Autodesk Fusion 360 part; units mm, degrees
(part 4 of 11)
  line L2513 (1.92, -15.2997) -> (1.92, -13.2625)
  arc A163 (1.92, -13.2625) -> (1.2372, -12.9797) centre (1.52, -13.2625) ccw
  line L2514 (1.2372, -12.9797) -> (-0.0459, -14.2627)
  line L2515 (-0.0459, -14.2627) -> (-0.0798, -14.2989)
  line L2516 (-0.0798, -14.2989) -> (-0.1133, -14.3397)
  line L2517 (-0.1133, -14.3397) -> (-0.1441, -14.3827)
  line L2518 (-0.1441, -14.3827) -> (-0.172, -14.4275)
  line L2519 (-0.172, -14.4275) -> (-0.1969, -14.4741)
  line L2520 (-0.1969, -14.4741) -> (-0.2187, -14.5222)
  line L2521 (-0.2187, -14.5222) -> (-0.2373, -14.5717)
  line L2522 (-0.2373, -14.5717) -> (-0.2526, -14.6222)
  line L2523 (-0.2526, -14.6222) -> (-0.2646, -14.6736)
  line L2524 (-0.2646, -14.6736) -> (-0.2732, -14.7258)
  line L2525 (-0.2732, -14.7258) -> (-0.2786, -14.7804)
  line L2526 (-0.2786, -14.7804) -> (-0.28, -14.8985)
  line L2527 (-0.28, -14.8985) -> (-0.28, -25.1009)
  line L2528 (-0.28, -25.1009) -> (-0.2786, -25.2189)
  line L2529 (-0.2786, -25.2189) -> (-0.2732, -25.2736)
  line L2530 (-0.2732, -25.2736) -> (-0.2646, -25.3257)
  line L2531 (-0.2646, -25.3257) -> (-0.2526, -25.3771)
  line L2532 (-0.2526, -25.3771) -> (-0.2373, -25.4277)
  line L2533 (-0.2373, -25.4277) -> (-0.2187, -25.4771)
  line L2534 (-0.2187, -25.4771) -> (-0.1969, -25.5252)
  line L2535 (-0.1969, -25.5252) -> (-0.172, -25.5718)
  line L2536 (-0.172, -25.5718) -> (-0.1441, -25.6166)
  line L2537 (-0.1441, -25.6166) -> (-0.1133, -25.6596)
  line L2538 (-0.1133, -25.6596) -> (-0.0798, -25.7004)
  line L2539 (-0.0798, -25.7004) -> (-0.0459, -25.7366)
  line L2540 (-0.0459, -25.7366) -> (1.2372, -27.0197)
  arc A164 (1.2372, -27.0197) -> (1.92, -26.7368) centre (1.52, -26.7368) ccw
  line L2541 (1.92, -26.7368) -> (1.92, -24.6997)
  line L2542 (1.92, -24.6997) -> (3.2765, -24.6997)
  line L2543 (3.2765, -24.6997) -> (5.82, -27.2432)
  line L2544 (5.82, -27.2432) -> (5.82, -29.8826)
  line L2545 (5.82, -29.8826) -> (5.937, -29.9997)
  line L2546 (5.937, -29.9997) -> (5.82, -30.1167)
  line L2547 (5.82, -30.1167) -> (5.82, -32.7562)
  line L2548 (5.82, -32.7562) -> (3.2765, -35.2997)
  line L2549 (3.2765, -35.2997) -> (1.92, -35.2997)
  line L2550 (1.92, -35.2997) -> (1.92, -33.2625)
  arc A165 (1.92, -33.2625) -> (1.2372, -32.9797) centre (1.52, -33.2625) ccw
  line L2551 (1.2372, -32.9797) -> (-0.0459, -34.2627)
  line L2552 (-0.0459, -34.2627) -> (-0.0798, -34.2989)
  line L2553 (-0.0798, -34.2989) -> (-0.1133, -34.3397)
  line L2554 (-0.1133, -34.3397) -> (-0.1441, -34.3827)
  line L2555 (-0.1441, -34.3827) -> (-0.172, -34.4275)
  line L2556 (-0.172, -34.4275) -> (-0.1969, -34.4741)
  line L2557 (-0.1969, -34.4741) -> (-0.2187, -34.5222)
  line L2558 (-0.2187, -34.5222) -> (-0.2373, -34.5717)
  line L2559 (-0.2373, -34.5717) -> (-0.2526, -34.6222)
  line L2560 (-0.2526, -34.6222) -> (-0.2646, -34.6736)
  line L2561 (-0.2646, -34.6736) -> (-0.2732, -34.7258)
  line L2562 (-0.2732, -34.7258) -> (-0.2786, -34.7804)
  line L2563 (-0.2786, -34.7804) -> (-0.28, -34.8985)
  line L2564 (-0.28, -34.8985) -> (-0.28, -45.1009)
  line L2565 (-0.28, -45.1009) -> (-0.2786, -45.2189)
  line L2566 (-0.2786, -45.2189) -> (-0.2732, -45.2736)
  line L2567 (-0.2732, -45.2736) -> (-0.2646, -45.3257)
  line L2568 (-0.2646, -45.3257) -> (-0.2526, -45.3771)
  line L2569 (-0.2526, -45.3771) -> (-0.2373, -45.4277)
  line L2570 (-0.2373, -45.4277) -> (-0.2187, -45.4771)
  line L2571 (-0.2187, -45.4771) -> (-0.1969, -45.5252)
  line L2572 (-0.1969, -45.5252) -> (-0.172, -45.5718)
  line L2573 (-0.172, -45.5718) -> (-0.1441, -45.6166)
  line L2574 (-0.1441, -45.6166) -> (-0.1133, -45.6596)
  line L2575 (-0.1133, -45.6596) -> (-0.0798, -45.7004)
  line L2576 (-0.0798, -45.7004) -> (-0.0459, -45.7366)
  line L2577 (-0.0459, -45.7366) -> (1.2372, -47.0197)
  arc A166 (1.2372, -47.0197) -> (1.92, -46.7368) centre (1.52, -46.7368) ccw
  line L2578 (1.92, -46.7368) -> (1.92, -44.6997)
  line L2579 (1.92, -44.6997) -> (3.2765, -44.6997)
  line L2580 (3.2765, -44.6997) -> (5.82, -47.2432)
  line L2581 (5.82, -47.2432) -> (5.82, -49.8826)
  line L2582 (5.82, -49.8826) -> (5.937, -49.9997)
  line L2583 (5.937, -49.9997) -> (5.82, -50.1167)
  line L2584 (5.82, -50.1167) -> (5.82, -52.7562)
  line L2585 (5.82, -52.7562) -> (3.2765, -55.2997)
  line L2586 (3.2765, -55.2997) -> (1.92, -55.2997)
  line L2587 (1.92, -55.2997) -> (1.92, -53.2625)
  arc A167 (1.92, -53.2625) -> (1.2372, -52.9797) centre (1.52, -53.2625) ccw
  line L2588 (1.2372, -52.9797) -> (-0.0459, -54.2627)
  line L2589 (-0.0459, -54.2627) -> (-0.0798, -54.2989)
  line L2590 (-0.0798, -54.2989) -> (-0.1133, -54.3397)
  line L2591 (-0.1133, -54.3397) -> (-0.1441, -54.3827)
  line L2592 (-0.1441, -54.3827) -> (-0.172, -54.4275)
  line L2593 (-0.172, -54.4275) -> (-0.1969, -54.4741)
  line L2594 (-0.1969, -54.4741) -> (-0.2187, -54.5222)
  line L2595 (-0.2187, -54.5222) -> (-0.2373, -54.5717)
  line L2596 (-0.2373, -54.5717) -> (-0.2526, -54.6222)
  line L2597 (-0.2526, -54.6222) -> (-0.2646, -54.6736)
  line L2598 (-0.2646, -54.6736) -> (-0.2732, -54.7258)
  line L2599 (-0.2732, -54.7258) -> (-0.2786, -54.7804)
  line L2600 (-0.2786, -54.7804) -> (-0.28, -54.8985)
  line L2601 (-0.28, -54.8985) -> (-0.28, -65.1009)
  line L2602 (-0.28, -65.1009) -> (-0.2786, -65.2189)
  line L2603 (-0.2786, -65.2189) -> (-0.2732, -65.2736)
  line L2604 (-0.2732, -65.2736) -> (-0.2646, -65.3257)
  line L2605 (-0.2646, -65.3257) -> (-0.2526, -65.3771)
  line L2606 (-0.2526, -65.3771) -> (-0.2373, -65.4277)
  line L2607 (-0.2373, -65.4277) -> (-0.2187, -65.4771)
  line L2608 (-0.2187, -65.4771) -> (-0.1969, -65.5252)
  line L2609 (-0.1969, -65.5252) -> (-0.172, -65.5718)
  line L2610 (-0.172, -65.5718) -> (-0.1441, -65.6166)
  line L2611 (-0.1441, -65.6166) -> (-0.1133, -65.6596)
  line L2612 (-0.1133, -65.6596) -> (-0.0798, -65.7004)
  line L2613 (-0.0798, -65.7004) -> (-0.0459, -65.7366)
  line L2614 (-0.0459, -65.7366) -> (1.2372, -67.0197)
  arc A168 (1.2372, -67.0197) -> (1.92, -66.7368) centre (1.52, -66.7368) ccw
  line L2615 (1.92, -66.7368) -> (1.92, -64.6997)
  line L2616 (1.92, -64.6997) -> (3.2765, -64.6997)
  line L2617 (3.2765, -64.6997) -> (5.82, -67.2432)
  line L2618 (5.82, -67.2432) -> (5.82, -69.8826)
  line L2619 (5.82, -69.8826) -> (5.937, -69.9997)
  line L2620 (5.937, -69.9997) -> (5.82, -70.1167)
  line L2621 (5.82, -70.1167) -> (5.82, -72.7562)
  line L2622 (5.82, -72.7562) -> (3.2765, -75.2997)
  line L2623 (3.2765, -75.2997) -> (1.92, -75.2997)
  line L2624 (1.92, -75.2997) -> (1.92, -73.2625)
  arc A169 (1.92, -73.2625) -> (1.2372, -72.9797) centre (1.52, -73.2625) ccw
  line L2625 (1.2372, -72.9797) -> (-0.0459, -74.2627)
  line L2626 (-0.0459, -74.2627) -> (-0.0798, -74.2989)
  line L2627 (-0.0798, -74.2989) -> (-0.1133, -74.3397)
  line L2628 (-0.1133, -74.3397) -> (-0.1441, -74.3827)
  line L2629 (-0.1441, -74.3827) -> (-0.172, -74.4275)
  line L2630 (-0.172, -74.4275) -> (-0.1969, -74.4741)
  line L2631 (-0.1969, -74.4741) -> (-0.2187, -74.5222)
  line L2632 (-0.2187, -74.5222) -> (-0.2373, -74.5717)
  line L2633 (-0.2373, -74.5717) -> (-0.2526, -74.6222)
  line L2634 (-0.2526, -74.6222) -> (-0.2646, -74.6736)
  line L2635 (-0.2646, -74.6736) -> (-0.2732, -74.7258)
  line L2636 (-0.2732, -74.7258) -> (-0.2786, -74.7804)
  line L2637 (-0.2786, -74.7804) -> (-0.28, -74.8985)
  line L2638 (-0.28, -74.8985) -> (-0.28, -78.4997)
  line L2639 (-0.28, -78.4997) -> (-0.28, -79.4997)
  arc A170 (-0.28, -79.4997) -> (0.42, -80.1997) centre (0.42, -79.4997) ccw
  line L2640 (0.42, -80.1997) -> (1.42, -80.1997)
  line L2641 (1.42, -80.1997) -> (5.0918, -80.1997)
  line L2642 (5.0918, -80.1997) -> (5.1413, -80.198)
  line L2643 (5.1413, -80.198) -> (5.1939, -80.1929)
  line L2644 (5.1939, -80.1929) -> (5.246, -80.1843)
  line L2645 (5.246, -80.1843) -> (5.2975, -80.1723)
  line L2646 (5.2975, -80.1723) -> (5.348, -80.1569)
  line L2647 (5.348, -80.1569) -> (5.3974, -80.1383)
  line L2648 (5.3974, -80.1383) -> (5.4455, -80.1165)
  line L2649 (5.4455, -80.1165) -> (5.4921, -80.0916)
  line L2650 (5.4921, -80.0916) -> (5.537, -80.0637)
  line L2651 (5.537, -80.0637) -> (5.5799, -80.033)
  line L2652 (5.5799, -80.033) -> (5.6207, -79.9995)
  line L2653 (5.6207, -79.9995) -> (5.6569, -79.9656)
  line L2654 (5.6569, -79.9656) -> (6.94, -78.6825)
  arc A171 (6.94, -78.6825) -> (6.6572, -77.9997) centre (6.6572, -78.3997) ccw
  line L2655 (6.6572, -77.9997) -> (4.62, -77.9997)
  line L2656 (4.62, -77.9997) -> (4.62, -76.6432)
  line L2657 (4.62, -76.6432) -> (7.1635, -74.0997)
  line L2658 (7.1635, -74.0997) -> (9.7981, -74.0997)
  line L2659 (9.7981, -74.0997) -> (9.9208, -73.977)
  line L2660 (9.9208, -73.977) -> (10.0448, -74.0997)
  line L2661 (10.0448, -74.0997) -> (12.6765, -74.0997)
  line L2662 (12.6765, -74.0997) -> (15.22, -76.6432)
  line L2663 (15.22, -76.6432) -> (15.22, -77.9997)
  line L2664 (15.22, -77.9997) -> (13.1828, -77.9997)
  arc A172 (13.1828, -77.9997) -> (12.9, -78.6825) centre (13.1828, -78.3997) ccw
  line L2665 (12.9, -78.6825) -> (14.1831, -79.9656)
  line L2666 (14.1831, -79.9656) -> (14.2193, -79.9995)
  line L2667 (14.2193, -79.9995) -> (14.2601, -80.033)
  line L2668 (14.2601, -80.033) -> (14.303, -80.0637)
  line L2669 (14.303, -80.0637) -> (14.3479, -80.0916)
  line L2670 (14.3479, -80.0916) -> (14.3945, -80.1165)
  line L2671 (14.3945, -80.1165) -> (14.4426, -80.1383)
  line L2672 (14.4426, -80.1383) -> (14.492, -80.1569)
  line L2673 (14.492, -80.1569) -> (14.5425, -80.1723)
  line L2674 (14.5425, -80.1723) -> (14.594, -80.1843)
  line L2675 (14.594, -80.1843) -> (14.6461, -80.1929)
  line L2676 (14.6461, -80.1929) -> (14.6987, -80.198)
  line L2677 (14.6987, -80.198) -> (14.7482, -80.1997)
  line L2678 (14.7482, -80.1997) -> (18.42, -80.1997)
  line L2679 (18.42, -80.1997) -> (19.42, -80.1997)
  arc A173 (19.42, -80.1997) -> (20.12, -79.4997) centre (19.42, -79.4997) ccw
  line L2680 (20.12, -79.4997) -> (20.12, -78.4997)
  line L2681 (20.12, -78.4997) -> (20.12, -74.8278)
  line L2682 (20.12, -74.8278) -> (20.1184, -74.7783)
  line L2683 (20.1184, -74.7783) -> (20.1132, -74.7258)
  line L2684 (20.1132, -74.7258) -> (20.1046, -74.6736)
  line L2685 (20.1046, -74.6736) -> (20.0926, -74.6222)
  line L2686 (20.0926, -74.6222) -> (20.0773, -74.5717)
  line L2687 (20.0773, -74.5717) -> (20.0587, -74.5222)
  line L2688 (20.0587, -74.5222) -> (20.0369, -74.4741)
  line L2689 (20.0369, -74.4741) -> (20.012, -74.4275)
  line L2690 (20.012, -74.4275) -> (19.9841, -74.3827)
  line L2691 (19.9841, -74.3827) -> (19.9533, -74.3397)
  line L2692 (19.9533, -74.3397) -> (19.9198, -74.2989)
  line L2693 (19.9198, -74.2989) -> (19.8859, -74.2627)
  line L2694 (19.8859, -74.2627) -> (18.6028, -72.9797)
  arc A174 (18.6028, -72.9797) -> (17.92, -73.2625) centre (18.32, -73.2625) ccw
  line L2695 (17.92, -73.2625) -> (17.92, -75.2997)
  line L2696 (17.92, -75.2997) -> (16.5635, -75.2997)
  line L2697 (16.5635, -75.2997) -> (14.02, -72.7562)
  line L2698 (14.02, -72.7562) -> (14.02, -70.1167)
  line L2699 (14.02, -70.1167) -> (13.903, -69.9997)
  line L2700 (13.903, -69.9997) -> (14.02, -69.8826)
  line L2701 (14.02, -69.8826) -> (14.02, -67.2432)
  line L2702 (14.02, -67.2432) -> (16.5635, -64.6997)
  line L2703 (16.5635, -64.6997) -> (17.92, -64.6997)
  line L2704 (17.92, -64.6997) -> (17.92, -66.7368)
  arc A175 (17.92, -66.7368) -> (18.6028, -67.0197) centre (18.32, -66.7368) ccw
  line L2705 (18.6028, -67.0197) -> (19.8859, -65.7366)
  line L2706 (19.8859, -65.7366) -> (19.9198, -65.7004)
  line L2707 (19.9198, -65.7004) -> (19.9533, -65.6596)
  line L2708 (19.9533, -65.6596) -> (19.9841, -65.6166)
  line L2709 (19.9841, -65.6166) -> (20.012, -65.5718)
  line L2710 (20.012, -65.5718) -> (20.0369, -65.5252)
  line L2711 (20.0369, -65.5252) -> (20.0587, -65.4771)
  line L2712 (20.0587, -65.4771) -> (20.0773, -65.4277)
  line L2713 (20.0773, -65.4277) -> (20.0926, -65.3771)
  line L2714 (20.0926, -65.3771) -> (20.1046, -65.3257)
  line L2715 (20.1046, -65.3257) -> (20.1132, -65.2736)
  line L2716 (20.1132, -65.2736) -> (20.1186, -65.2189)
  line L2717 (20.1186, -65.2189) -> (20.12, -65.1009)
  line L2718 (20.12, -65.1009) -> (20.12, -54.8985)
  line L2719 (20.12, -54.8985) -> (20.1186, -54.7804)
  line L2720 (20.1186, -54.7804) -> (20.1132, -54.7258)
  line L2721 (20.1132, -54.7258) -> (20.1046, -54.6736)
  line L2722 (20.1046, -54.6736) -> (20.0926, -54.6222)
  line L2723 (20.0926, -54.6222) -> (20.0773, -54.5717)
  line L2724 (20.0773, -54.5717) -> (20.0587, -54.5222)
  line L2725 (20.0587, -54.5222) -> (20.0369, -54.4741)
  line L2726 (20.0369, -54.4741) -> (20.012, -54.4275)
  line L2727 (20.012, -54.4275) -> (19.9841, -54.3827)
  line L2728 (19.9841, -54.3827) -> (19.9533, -54.3397)
  line L2729 (19.9533, -54.3397) -> (19.9198, -54.2989)
  line L2730 (19.9198, -54.2989) -> (19.8859, -54.2627)
  line L2731 (19.8859, -54.2627) -> (18.6028, -52.9797)
  arc A176 (18.6028, -52.9797) -> (17.92, -53.2625) centre (18.32, -53.2625) ccw
  line L2732 (17.92, -53.2625) -> (17.92, -55.2997)
  line L2733 (17.92, -55.2997) -> (16.5635, -55.2997)
  line L2734 (16.5635, -55.2997) -> (14.02, -52.7562)
  line L2735 (14.02, -52.7562) -> (14.02, -50.1167)
  line L2736 (14.02, -50.1167) -> (13.903, -49.9997)
  line L2737 (13.903, -49.9997) -> (14.02, -49.8826)
  line L2738 (14.02, -49.8826) -> (14.02, -47.2432)
  line L2739 (14.02, -47.2432) -> (16.5635, -44.6997)
  line L2740 (16.5635, -44.6997) -> (17.92, -44.6997)
  line L2741 (17.92, -44.6997) -> (17.92, -46.7368)
  arc A177 (17.92, -46.7368) -> (18.6028, -47.0197) centre (18.32, -46.7368) ccw
  line L2742 (18.6028, -47.0197) -> (19.8859, -45.7366)
  line L2743 (19.8859, -45.7366) -> (19.9198, -45.7004)
  line L2744 (19.9198, -45.7004) -> (19.9533, -45.6596)
  line L2745 (19.9533, -45.6596) -> (19.9841, -45.6166)
  line L2746 (19.9841, -45.6166) -> (20.012, -45.5718)
  line L2747 (20.012, -45.5718) -> (20.0369, -45.5252)
  line L2748 (20.0369, -45.5252) -> (20.0587, -45.4771)
  line L2749 (20.0587, -45.4771) -> (20.0773, -45.4277)
  line L2750 (20.0773, -45.4277) -> (20.0926, -45.3771)
  line L2751 (20.0926, -45.3771) -> (20.1046, -45.3257)
  line L2752 (20.1046, -45.3257) -> (20.1132, -45.2736)
  line L2753 (20.1132, -45.2736) -> (20.1186, -45.2189)
  line L2754 (20.1186, -45.2189) -> (20.12, -45.1009)
  line L2755 (20.12, -45.1009) -> (20.12, -34.8985)
  line L2756 (20.12, -34.8985) -> (20.1186, -34.7804)
  line L2757 (20.1186, -34.7804) -> (20.1132, -34.7258)
  line L2758 (20.1132, -34.7258) -> (20.1046, -34.6736)
  line L2759 (20.1046, -34.6736) -> (20.0926, -34.6222)
  line L2760 (20.0926, -34.6222) -> (20.0773, -34.5717)
  line L2761 (20.0773, -34.5717) -> (20.0587, -34.5222)
  line L2762 (20.0587, -34.5222) -> (20.0369, -34.4741)
  line L2763 (20.0369, -34.4741) -> (20.012, -34.4275)
  line L2764 (20.012, -34.4275) -> (19.9841, -34.3827)
  line L2765 (19.9841, -34.3827) -> (19.9533, -34.3397)
  line L2766 (19.9533, -34.3397) -> (19.9198, -34.2989)
  line L2767 (19.9198, -34.2989) -> (19.8859, -34.2627)
  line L2768 (19.8859, -34.2627) -> (18.6028, -32.9797)
  arc A178 (18.6028, -32.9797) -> (17.92, -33.2625) centre (18.32, -33.2625) ccw
  line L2769 (17.92, -33.2625) -> (17.92, -35.2997)
  line L2770 (17.92, -35.2997) -> (16.5635, -35.2997)
  line L2771 (16.5635, -35.2997) -> (14.02, -32.7562)
  line L2772 (14.02, -32.7562) -> (14.02, -30.1167)
  line L2773 (14.02, -30.1167) -> (13.903, -29.9997)
  line L2774 (13.903, -29.9997) -> (14.02, -29.8826)
  line L2775 (14.02, -29.8826) -> (14.02, -27.2432)
  line L2776 (14.02, -27.2432) -> (16.5635, -24.6997)
  line L2777 (16.5635, -24.6997) -> (17.92, -24.6997)
  line L2778 (17.92, -24.6997) -> (17.92, -26.7368)
  arc A179 (17.92, -26.7368) -> (18.6028, -27.0197) centre (18.32, -26.7368) ccw
  line L2779 (18.6028, -27.0197) -> (19.8859, -25.7366)
  line L2780 (19.8859, -25.7366) -> (19.9198, -25.7004)
  line L2781 (19.9198, -25.7004) -> (19.9533, -25.6596)
  line L2782 (19.9533, -25.6596) -> (19.9841, -25.6166)
  line L2783 (19.9841, -25.6166) -> (20.012, -25.5718)
  line L2784 (20.012, -25.5718) -> (20.0369, -25.5252)
  line L2785 (20.0369, -25.5252) -> (20.0587, -25.4771)
  line L2786 (20.0587, -25.4771) -> (20.0773, -25.4277)
  line L2787 (20.0773, -25.4277) -> (20.0926, -25.3771)
  line L2788 (20.0926, -25.3771) -> (20.1046, -25.3257)
  line L2789 (20.1046, -25.3257) -> (20.1132, -25.2736)
  line L2790 (20.1132, -25.2736) -> (20.1186, -25.2189)
  line L2791 (20.1186, -25.2189) -> (20.12, -25.1009)
  line L2792 (20.12, -25.1009) -> (20.12, -14.8985)
  line L2793 (20.12, -14.8985) -> (20.1186, -14.7804)
  line L2794 (20.1186, -14.7804) -> (20.1132, -14.7258)
  line L2795 (20.1132, -14.7258) -> (20.1046, -14.6736)
  line L2796 (20.1046, -14.6736) -> (20.0926, -14.6222)
  line L2797 (20.0926, -14.6222) -> (20.0773, -14.5717)
  line L2798 (20.0773, -14.5717) -> (20.0587, -14.5222)
  line L2799 (20.0587, -14.5222) -> (20.0369, -14.4741)
  line L2800 (20.0369, -14.4741) -> (20.012, -14.4275)
  line L2801 (20.012, -14.4275) -> (19.9841, -14.3827)
  line L2802 (19.9841, -14.3827) -> (19.9533, -14.3397)
  line L2803 (19.9533, -14.3397) -> (19.9198, -14.2989)
  line L2804 (19.9198, -14.2989) -> (19.8859, -14.2627)
  line L2805 (19.8859, -14.2627) -> (18.6028, -12.9797)
  arc A180 (18.6028, -12.9797) -> (17.92, -13.2625) centre (18.32, -13.2625) ccw
  line L2806 (17.92, -13.2625) -> (17.92, -15.2997)
  line L2807 (17.92, -15.2997) -> (16.5635, -15.2997)
  line L2808 (16.5635, -15.2997) -> (14.02, -12.7562)
  line L2809 (14.02, -12.7562) -> (14.02, -10.1167)
  line L2810 (14.02, -10.1167) -> (13.903, -9.9997)
  line L2811 (13.903, -9.9997) -> (14.02, -9.8826)
  line L2812 (14.02, -9.8826) -> (14.02, -7.2432)
  line L2813 (14.02, -7.2432) -> (16.5635, -4.6997)
  line L2814 (16.5635, -4.6997) -> (17.92, -4.6997)
  line L2815 (17.92, -4.6997) -> (17.92, -6.7368)
  arc A181 (17.92, -6.7368) -> (18.6028, -7.0197) centre (18.32, -6.7368) ccw
  line L2816 (18.6028, -7.0197) -> (19.8859, -5.7366)
  line L2817 (19.8859, -5.7366) -> (19.9198, -5.7004)
  line L2818 (9.92, -13.9755) -> (10.0441, -14.0997)
  line L2819 (10.0441, -14.0997) -> (12.6765, -14.0997)
  line L2820 (12.6765, -14.0997) -> (16.0765, -17.4997)
  line L2821 (16.0765, -17.4997) -> (17.92, -17.4997)
  line L2822 (17.92, -17.4997) -> (17.92, -22.4997)
  line L2823 (17.92, -22.4997) -> (16.0765, -22.4997)
  line L2824 (16.0765, -22.4997) -> (12.6765, -25.8997)
  line L2825 (12.6765, -25.8997) -> (10.0441, -25.8997)
  line L2826 (10.0441, -25.8997) -> (9.92, -26.0238)
  line L2827 (9.92, -26.0238) -> (9.7959, -25.8997)
  line L2828 (9.7959, -25.8997) -> (7.1635, -25.8997)
  line L2829 (7.1635, -25.8997) -> (3.7635, -22.4997)
  line L2830 (3.7635, -22.4997) -> (1.92, -22.4997)
  line L2831 (1.92, -22.4997) -> (1.92, -17.4997)
  line L2832 (1.92, -17.4997) -> (3.7635, -17.4997)
  line L2833 (3.7635, -17.4997) -> (7.1635, -14.0997)
  line L2834 (7.1635, -14.0997) -> (9.7959, -14.0997)
  line L2835 (9.7959, -14.0997) -> (9.92, -13.9755)
  line L2836 (9.92, -33.9755) -> (10.0441, -34.0997)
  line L2837 (10.0441, -34.0997) -> (12.6765, -34.0997)
  line L2838 (12.6765, -34.0997) -> (16.0765, -37.4997)
  line L2839 (16.0765, -37.4997) -> (17.92, -37.4997)
  line L2840 (17.92, -37.4997) -> (17.92, -42.4997)
  line L2841 (17.92, -42.4997) -> (16.0765, -42.4997)
  line L2842 (16.0765, -42.4997) -> (12.6765, -45.8997)
  line L2843 (12.6765, -45.8997) -> (10.0441, -45.8997)
  line L2844 (10.0441, -45.8997) -> (9.92, -46.0238)
  line L2845 (9.92, -46.0238) -> (9.7959, -45.8997)
  line L2846 (9.7959, -45.8997) -> (7.1635, -45.8997)
  line L2847 (7.1635, -45.8997) -> (3.7635, -42.4997)
  line L2848 (3.7635, -42.4997) -> (1.92, -42.4997)
  line L2849 (1.92, -42.4997) -> (1.92, -37.4997)
  line L2850 (1.92, -37.4997) -> (3.7635, -37.4997)
  line L2851 (3.7635, -37.4997) -> (7.1635, -34.0997)
  line L2852 (7.1635, -34.0997) -> (9.7959, -34.0997)
  line L2853 (9.7959, -34.0997) -> (9.92, -33.9755)
  line L2854 (16.0765, -57.4997) -> (17.92, -57.4997)
  line L2855 (17.92, -57.4997) -> (17.92, -62.4997)
  line L2856 (17.92, -62.4997) -> (16.0765, -62.4997)
  line L2857 (16.0765, -62.4997) -> (12.6765, -65.8997)
  line L2858 (12.6765, -65.8997) -> (10.0441, -65.8997)
  line L2859 (10.0441, -65.8997) -> (9.92, -66.0238)
  line L2860 (9.92, -66.0238) -> (9.7959, -65.8997)
  line L2861 (9.7959, -65.8997) -> (7.1635, -65.8997)
  line L2862 (7.1635, -65.8997) -> (3.7635, -62.4997)
  line L2863 (3.7635, -62.4997) -> (1.92, -62.4997)
  line L2864 (1.92, -62.4997) -> (1.92, -57.4997)
  line L2865 (1.92, -57.4997) -> (3.7635, -57.4997)
  line L2866 (3.7635, -57.4997) -> (7.1635, -54.0997)
  line L2867 (7.1635, -54.0997) -> (9.7959, -54.0997)
  line L2868 (9.7959, -54.0997) -> (9.92, -53.9755)
  line L2869 (9.92, -53.9755) -> (10.0441, -54.0997)
  line L2870 (10.0441, -54.0997) -> (12.6765, -54.0997)
  line L2871 (12.6765, -54.0997) -> (16.0765, -57.4997)
  line L2872 (9.92, -86.0238) -> (9.7959, -85.8997)
  line L2873 (9.7959, -85.8997) -> (7.1635, -85.8997)
  line L2874 (7.1635, -85.8997) -> (4.62, -83.3562)
  line L2875 (4.62, -83.3562) -> (4.62, -81.9997)
  line L2876 (4.62, -81.9997) -> (6.6572, -81.9997)
  arc A182 (6.6572, -81.9997) -> (6.94, -81.3168) centre (6.6572, -81.5997) ccw
  line L2877 (6.94, -81.3168) -> (5.6569, -80.0337)
  line L2878 (5.6569, -80.0337) -> (5.6207, -79.9999)
  line L2879 (5.6207, -79.9999) -> (5.5799, -79.9663)
  line L2880 (5.5799, -79.9663) -> (5.537, -79.9356)
  line L2881 (5.537, -79.9356) -> (5.4921, -79.9077)
  line L2882 (5.4921, -79.9077) -> (5.4455, -79.8828)
  line L2883 (5.4455, -79.8828) -> (5.3974, -79.861)
  line L2884 (5.3974, -79.861) -> (5.348, -79.8424)
  line L2885 (5.348, -79.8424) -> (5.2975, -79.8271)
  line L2886 (5.2975, -79.8271) -> (5.246, -79.8151)
  line L2887 (5.246, -79.8151) -> (5.1939, -79.8065)
  line L2888 (5.1939, -79.8065) -> (5.1413, -79.8013)
  line L2889 (5.1413, -79.8013) -> (5.0918, -79.7997)
  line L2890 (5.0918, -79.7997) -> (1.42, -79.7997)
  line L2891 (1.42, -79.7997) -> (0.42, -79.7997)
  arc A183 (0.42, -79.7997) -> (-0.28, -80.4997) centre (0.42, -80.4997) ccw
  line L2892 (-0.28, -80.4997) -> (-0.28, -81.4997)
  line L2893 (-0.28, -81.4997) -> (-0.28, -85.1009)
  line L2894 (-0.28, -85.1009) -> (-0.2786, -85.2189)
  line L2895 (-0.2786, -85.2189) -> (-0.2732, -85.2736)
  line L2896 (-0.2732, -85.2736) -> (-0.2646, -85.3257)
  line L2897 (-0.2646, -85.3257) -> (-0.2526, -85.3771)
  line L2898 (-0.2526, -85.3771) -> (-0.2373, -85.4277)
  line L2899 (-0.2373, -85.4277) -> (-0.2187, -85.4771)
  line L2900 (-0.2187, -85.4771) -> (-0.1969, -85.5252)
  line L2901 (-0.1969, -85.5252) -> (-0.172, -85.5718)
  line L2902 (-0.172, -85.5718) -> (-0.1441, -85.6166)
  line L2903 (-0.1441, -85.6166) -> (-0.1133, -85.6596)
  line L2904 (-0.1133, -85.6596) -> (-0.0798, -85.7004)
  line L2905 (-0.0798, -85.7004) -> (-0.0459, -85.7366)
  line L2906 (-0.0459, -85.7366) -> (1.2372, -87.0197)
  arc A184 (1.2372, -87.0197) -> (1.92, -86.7368) centre (1.52, -86.7368) ccw
  line L2907 (1.92, -86.7368) -> (1.92, -84.6997)
  line L2908 (1.92, -84.6997) -> (3.2765, -84.6997)
  line L2909 (3.2765, -84.6997) -> (5.82, -87.2432)
  line L2910 (5.82, -87.2432) -> (5.82, -89.8826)
  line L2911 (5.82, -89.8826) -> (5.937, -89.9997)
  line L2912 (5.937, -89.9997) -> (5.82, -90.1167)
  line L2913 (5.82, -90.1167) -> (5.82, -92.7562)
  line L2914 (5.82, -92.7562) -> (3.2765, -95.2997)
  line L2915 (3.2765, -95.2997) -> (1.92, -95.2997)
  line L2916 (1.92, -95.2997) -> (1.92, -93.2625)
  arc A185 (1.92, -93.2625) -> (1.2372, -92.9797) centre (1.52, -93.2625) ccw
  line L2917 (1.2372, -92.9797) -> (-0.0459, -94.2627)
  line L2918 (-0.0459, -94.2627) -> (-0.0798, -94.2989)
  line L2919 (-0.0798, -94.2989) -> (-0.1133, -94.3397)
  line L2920 (-0.1133, -94.3397) -> (-0.1441, -94.3827)
  line L2921 (-0.1441, -94.3827) -> (-0.172, -94.4275)
  line L2922 (-0.172, -94.4275) -> (-0.1969, -94.4741)
  line L2923 (-0.1969, -94.4741) -> (-0.2187, -94.5222)
  line L2924 (-0.2187, -94.5222) -> (-0.2373, -94.5717)
  line L2925 (-0.2373, -94.5717) -> (-0.2526, -94.6222)
  line L2926 (-0.2526, -94.6222) -> (-0.2646, -94.6736)
  line L2927 (-0.2646, -94.6736) -> (-0.2732, -94.7258)
  line L2928 (-0.2732, -94.7258) -> (-0.2786, -94.7804)
  line L2929 (-0.2786, -94.7804) -> (-0.28, -94.8985)
  line L2930 (-0.28, -94.8985) -> (-0.28, -105.1009)
  line L2931 (-0.28, -105.1009) -> (-0.2786, -105.2189)
  line L2932 (-0.2786, -105.2189) -> (-0.2732, -105.2736)
  line L2933 (-0.2732, -105.2736) -> (-0.2646, -105.3257)
  line L2934 (-0.2646, -105.3257) -> (-0.2526, -105.3771)
  line L2935 (-0.2526, -105.3771) -> (-0.2373, -105.4277)
  line L2936 (-0.2373, -105.4277) -> (-0.2187, -105.4771)
  line L2937 (-0.2187, -105.4771) -> (-0.1969, -105.5252)
  line L2938 (-0.1969, -105.5252) -> (-0.172, -105.5718)
  line L2939 (-0.172, -105.5718) -> (-0.1441, -105.6166)
  line L2940 (-0.1441, -105.6166) -> (-0.1133, -105.6596)
  line L2941 (-0.1133, -105.6596) -> (-0.0798, -105.7004)
  line L2942 (-0.0798, -105.7004) -> (-0.0459, -105.7366)
  line L2943 (-0.0459, -105.7366) -> (1.2372, -107.0197)
  arc A186 (1.2372, -107.0197) -> (1.92, -106.7368) centre (1.52, -106.7368) ccw
  line L2944 (1.92, -106.7368) -> (1.92, -104.6997)
  line L2945 (1.92, -104.6997) -> (3.2765, -104.6997)
  line L2946 (3.2765, -104.6997) -> (5.82, -107.2432)
  line L2947 (5.82, -107.2432) -> (5.82, -109.8826)
  line L2948 (5.82, -109.8826) -> (5.937, -109.9997)
  line L2949 (5.937, -109.9997) -> (5.82, -110.1167)
  line L2950 (5.82, -110.1167) -> (5.82, -112.7562)
  line L2951 (5.82, -112.7562) -> (3.2765, -115.2997)
  line L2952 (3.2765, -115.2997) -> (1.92, -115.2997)
  line L2953 (1.92, -115.2997) -> (1.92, -113.2625)
  arc A187 (1.92, -113.2625) -> (1.2372, -112.9797) centre (1.52, -113.2625) ccw
  line L2954 (1.2372, -112.9797) -> (-0.0459, -114.2627)
  line L2955 (-0.0459, -114.2627) -> (-0.0798, -114.2989)
  line L2956 (-0.0798, -114.2989) -> (-0.1133, -114.3397)
  line L2957 (-0.1133, -114.3397) -> (-0.1441, -114.3827)
  line L2958 (-0.1441, -114.3827) -> (-0.172, -114.4275)
  line L2959 (-0.172, -114.4275) -> (-0.1969, -114.4741)
  line L2960 (-0.1969, -114.4741) -> (-0.2187, -114.5222)
  line L2961 (-0.2187, -114.5222) -> (-0.2373, -114.5717)
  line L2962 (-0.2373, -114.5717) -> (-0.2526, -114.6222)
  line L2963 (-0.2526, -114.6222) -> (-0.2646, -114.6736)
  line L2964 (-0.2646, -114.6736) -> (-0.2732, -114.7258)
  line L2965 (-0.2732, -114.7258) -> (-0.2786, -114.7804)
  line L2966 (-0.2786, -114.7804) -> (-0.28, -114.8985)
  line L2967 (-0.28, -114.8985) -> (-0.28, -125.1009)
  line L2968 (-0.28, -125.1009) -> (-0.2786, -125.2189)
  line L2969 (-0.2786, -125.2189) -> (-0.2732, -125.2736)
  line L2970 (-0.2732, -125.2736) -> (-0.2646, -125.3257)
  line L2971 (-0.2646, -125.3257) -> (-0.2526, -125.3771)
  line L2972 (-0.2526, -125.3771) -> (-0.2373, -125.4277)
  line L2973 (-0.2373, -125.4277) -> (-0.2187, -125.4771)
  line L2974 (-0.2187, -125.4771) -> (-0.1969, -125.5252)
  line L2975 (-0.1969, -125.5252) -> (-0.172, -125.5718)
  line L2976 (-0.172, -125.5718) -> (-0.1441, -125.6166)
  line L2977 (-0.1441, -125.6166) -> (-0.1133, -125.6596)
  line L2978 (-0.1133, -125.6596) -> (-0.0798, -125.7004)
  line L2979 (-0.0798, -125.7004) -> (-0.0459, -125.7366)
  line L2980 (-0.0459, -125.7366) -> (1.2372, -127.0197)
  arc A188 (1.2372, -127.0197) -> (1.92, -126.7368) centre (1.52, -126.7368) ccw
  line L2981 (1.92, -126.7368) -> (1.92, -124.6997)
  line L2982 (1.92, -124.6997) -> (3.2765, -124.6997)
  line L2983 (3.2765, -124.6997) -> (5.82, -127.2432)
  line L2984 (5.82, -127.2432) -> (5.82, -129.8826)
  line L2985 (5.82, -129.8826) -> (5.937, -129.9997)
  line L2986 (5.937, -129.9997) -> (5.82, -130.1167)
  line L2987 (5.82, -130.1167) -> (5.82, -132.7562)
  line L2988 (5.82, -132.7562) -> (3.2765, -135.2997)
  line L2989 (3.2765, -135.2997) -> (1.92, -135.2997)
  line L2990 (1.92, -135.2997) -> (1.92, -133.2625)
  arc A189 (1.92, -133.2625) -> (1.2372, -132.9797) centre (1.52, -133.2625) ccw
  line L2991 (1.2372, -132.9797) -> (-0.0459, -134.2627)
  line L2992 (-0.0459, -134.2627) -> (-0.0798, -134.2989)
  line L2993 (-0.0798, -134.2989) -> (-0.1133, -134.3397)
  line L2994 (-0.1133, -134.3397) -> (-0.1441, -134.3827)
  line L2995 (-0.1441, -134.3827) -> (-0.172, -134.4275)
  line L2996 (-0.172, -134.4275) -> (-0.1969, -134.4741)
  line L2997 (-0.1969, -134.4741) -> (-0.2187, -134.5222)
  line L2998 (-0.2187, -134.5222) -> (-0.2373, -134.5717)
  line L2999 (-0.2373, -134.5717) -> (-0.2526, -134.6222)
  line L3000 (-0.2526, -134.6222) -> (-0.2646, -134.6736)
  line L3001 (-0.2646, -134.6736) -> (-0.2732, -134.7258)
  line L3002 (-0.2732, -134.7258) -> (-0.2786, -134.7804)
  line L3003 (-0.2786, -134.7804) -> (-0.28, -134.8985)
  line L3004 (-0.28, -134.8985) -> (-0.28, -138.4997)
  line L3005 (-0.28, -138.4997) -> (-0.28, -139.4997)
  arc A190 (-0.28, -139.4997) -> (0.42, -140.1997) centre (0.42, -139.4997) ccw
  line L3006 (0.42, -140.1997) -> (1.42, -140.1997)
  line L3007 (1.42, -140.1997) -> (5.0918, -140.1997)
  line L3008 (5.0918, -140.1997) -> (5.1413, -140.198)
  line L3009 (5.1413, -140.198) -> (5.1939, -140.1929)
  line L3010 (5.1939, -140.1929) -> (5.246, -140.1843)
  line L3011 (5.246, -140.1843) -> (5.2975, -140.1723)
  line L3012 (5.2975, -140.1723) -> (5.348, -140.1569)
  line L3013 (5.348, -140.1569) -> (5.3974, -140.1383)
  line L3014 (5.3974, -140.1383) -> (5.4455, -140.1165)
  line L3015 (5.4455, -140.1165) -> (5.4921, -140.0916)
  line L3016 (5.4921, -140.0916) -> (5.537, -140.0637)
  line L3017 (5.537, -140.0637) -> (5.5799, -140.033)
  line L3018 (5.5799, -140.033) -> (5.6207, -139.9995)
  line L3019 (5.6207, -139.9995) -> (5.6569, -139.9656)
  line L3020 (5.6569, -139.9656) -> (6.94, -138.6825)
  arc A191 (6.94, -138.6825) -> (6.6572, -137.9997) centre (6.6572, -138.3997) ccw
  line L3021 (6.6572, -137.9997) -> (4.62, -137.9997)
  line L3022 (4.62, -137.9997) -> (4.62, -136.6432)
  line L3023 (4.62, -136.6432) -> (7.1635, -134.0997)
  line L3024 (7.1635, -134.0997) -> (9.7981, -134.0997)
  line L3025 (9.7981, -134.0997) -> (9.9208, -133.977)
  line L3026 (9.9208, -133.977) -> (10.0448, -134.0997)
  line L3027 (10.0448, -134.0997) -> (12.6765, -134.0997)
  line L3028 (12.6765, -134.0997) -> (15.22, -136.6432)
  line L3029 (15.22, -136.6432) -> (15.22, -137.9997)
  line L3030 (15.22, -137.9997) -> (13.1828, -137.9997)
  arc A192 (13.1828, -137.9997) -> (12.9, -138.6825) centre (13.1828, -138.3997) ccw
  line L3031 (12.9, -138.6825) -> (14.1831, -139.9656)
  line L3032 (14.1831, -139.9656) -> (14.2193, -139.9995)
  line L3033 (14.2193, -139.9995) -> (14.2601, -140.033)
  line L3034 (14.2601, -140.033) -> (14.303, -140.0637)
  line L3035 (14.303, -140.0637) -> (14.3479, -140.0916)
  line L3036 (14.3479, -140.0916) -> (14.3945, -140.1165)
  line L3037 (14.3945, -140.1165) -> (14.4426, -140.1383)
  line L3038 (14.4426, -140.1383) -> (14.492, -140.1569)
  line L3039 (14.492, -140.1569) -> (14.5425, -140.1723)
  line L3040 (14.5425, -140.1723) -> (14.594, -140.1843)
  line L3041 (14.594, -140.1843) -> (14.6461, -140.1929)
  line L3042 (14.6461, -140.1929) -> (14.6987, -140.198)
  line L3043 (14.6987, -140.198) -> (14.7482, -140.1997)
  line L3044 (14.7482, -140.1997) -> (18.42, -140.1997)
  line L3045 (18.42, -140.1997) -> (19.42, -140.1997)
  arc A193 (19.42, -140.1997) -> (20.12, -139.4997) centre (19.42, -139.4997) ccw
  line L3046 (20.12, -139.4997) -> (20.12, -138.4997)
  line L3047 (20.12, -138.4997) -> (20.12, -134.8278)
  line L3048 (20.12, -134.8278) -> (20.1184, -134.7783)
  line L3049 (20.1184, -134.7783) -> (20.1132, -134.7258)
  line L3050 (20.1132, -134.7258) -> (20.1046, -134.6736)
  line L3051 (20.1046, -134.6736) -> (20.0926, -134.6222)
  line L3052 (20.0926, -134.6222) -> (20.0773, -134.5717)
  line L3053 (20.0773, -134.5717) -> (20.0587, -134.5222)
  line L3054 (20.0587, -134.5222) -> (20.0369, -134.4741)
  line L3055 (20.0369, -134.4741) -> (20.012, -134.4275)
  line L3056 (20.012, -134.4275) -> (19.9841, -134.3827)
  line L3057 (19.9841, -134.3827) -> (19.9533, -134.3397)
  line L3058 (19.9533, -134.3397) -> (19.9198, -134.2989)
  line L3059 (19.9198, -134.2989) -> (19.8859, -134.2627)
  line L3060 (19.8859, -134.2627) -> (18.6028, -132.9797)
  arc A194 (18.6028, -132.9797) -> (17.92, -133.2625) centre (18.32, -133.2625) ccw
  line L3061 (17.92, -133.2625) -> (17.92, -135.2997)
  line L3062 (17.92, -135.2997) -> (16.5635, -135.2997)
  line L3063 (16.5635, -135.2997) -> (14.02, -132.7562)
  line L3064 (14.02, -132.7562) -> (14.02, -130.1167)
  line L3065 (14.02, -130.1167) -> (13.903, -129.9997)
  line L3066 (13.903, -129.9997) -> (14.02, -129.8826)
  line L3067 (14.02, -129.8826) -> (14.02, -127.2432)
  line L3068 (14.02, -127.2432) -> (16.5635, -124.6997)
  line L3069 (16.5635, -124.6997) -> (17.92, -124.6997)
  line L3070 (17.92, -124.6997) -> (17.92, -126.7368)
  arc A195 (17.92, -126.7368) -> (18.6028, -127.0197) centre (18.32, -126.7368) ccw
  line L3071 (18.6028, -127.0197) -> (19.8859, -125.7366)
  line L3072 (19.8859, -125.7366) -> (19.9198, -125.7004)
  line L3073 (19.9198, -125.7004) -> (19.9533, -125.6596)
  line L3074 (19.9533, -125.6596) -> (19.9841, -125.6166)
  line L3075 (19.9841, -125.6166) -> (20.012, -125.5718)
  line L3076 (20.012, -125.5718) -> (20.0369, -125.5252)
  line L3077 (20.0369, -125.5252) -> (20.0587, -125.4771)
  line L3078 (20.0587, -125.4771) -> (20.0773, -125.4277)
  line L3079 (20.0773, -125.4277) -> (20.0926, -125.3771)
  line L3080 (20.0926, -125.3771) -> (20.1046, -125.3257)
  line L3081 (20.1046, -125.3257) -> (20.1132, -125.2736)
  line L3082 (20.1132, -125.2736) -> (20.1186, -125.2189)
  line L3083 (20.1186, -125.2189) -> (20.12, -125.1009)
  line L3084 (20.12, -125.1009) -> (20.12, -114.8985)
  line L3085 (20.12, -114.8985) -> (20.1186, -114.7804)
  line L3086 (20.1186, -114.7804) -> (20.1132, -114.7258)
  line L3087 (20.1132, -114.7258) -> (20.1046, -114.6736)
  line L3088 (20.1046, -114.6736) -> (20.0926, -114.6222)
  line L3089 (20.0926, -114.6222) -> (20.0773, -114.5717)
  line L3090 (20.0773, -114.5717) -> (20.0587, -114.5222)
  line L3091 (20.0587, -114.5222) -> (20.0369, -114.4741)
  line L3092 (20.0369, -114.4741) -> (20.012, -114.4275)
  line L3093 (20.012, -114.4275) -> (19.9841, -114.3827)
  line L3094 (19.9841, -114.3827) -> (19.9533, -114.3397)
  line L3095 (19.9533, -114.3397) -> (19.9198, -114.2989)
  line L3096 (19.9198, -114.2989) -> (19.8859, -114.2627)
  line L3097 (19.8859, -114.2627) -> (18.6028, -112.9797)
  arc A196 (18.6028, -112.9797) -> (17.92, -113.2625) centre (18.32, -113.2625) ccw
  line L3098 (17.92, -113.2625) -> (17.92, -115.2997)
  line L3099 (17.92, -115.2997) -> (16.5635, -115.2997)
  line L3100 (16.5635, -115.2997) -> (14.02, -112.7562)
  line L3101 (14.02, -112.7562) -> (14.02, -110.1167)
  line L3102 (14.02, -110.1167) -> (13.903, -109.9997)
  line L3103 (13.903, -109.9997) -> (14.02, -109.8826)
  line L3104 (14.02, -109.8826) -> (14.02, -107.2432)
  line L3105 (14.02, -107.2432) -> (16.5635, -104.6997)
  line L3106 (16.5635, -104.6997) -> (17.92, -104.6997)
  line L3107 (17.92, -104.6997) -> (17.92, -106.7368)
  arc A197 (17.92, -106.7368) -> (18.6028, -107.0197) centre (18.32, -106.7368) ccw
  line L3108 (18.6028, -107.0197) -> (19.8859, -105.7366)
  line L3109 (19.8859, -105.7366) -> (19.9198, -105.7004)
  line L3110 (19.9198, -105.7004) -> (19.9533, -105.6596)
  line L3111 (19.9533, -105.6596) -> (19.9841, -105.6166)
  line L3112 (19.9841, -105.6166) -> (20.012, -105.5718)
  line L3113 (20.012, -105.5718) -> (20.0369, -105.5252)
  line L3114 (20.0369, -105.5252) -> (20.0587, -105.4771)
  line L3115 (20.0587, -105.4771) -> (20.0773, -105.4277)
  line L3116 (20.0773, -105.4277) -> (20.0926, -105.3771)
  line L3117 (20.0926, -105.3771) -> (20.1046, -105.3257)
  line L3118 (20.1046, -105.3257) -> (20.1132, -105.2736)
  line L3119 (20.1132, -105.2736) -> (20.1186, -105.2189)
  line L3120 (20.1186, -105.2189) -> (20.12, -105.1009)
  line L3121 (20.12, -105.1009) -> (20.12, -94.8985)
  line L3122 (20.12, -94.8985) -> (20.1186, -94.7804)
  line L3123 (20.1186, -94.7804) -> (20.1132, -94.7258)
  line L3124 (20.1132, -94.7258) -> (20.1046, -94.6736)
  line L3125 (20.1046, -94.6736) -> (20.0926, -94.6222)
  line L3126 (20.0926, -94.6222) -> (20.0773, -94.5717)
  line L3127 (20.0773, -94.5717) -> (20.0587, -94.5222)
  line L3128 (20.0587, -94.5222) -> (20.0369, -94.4741)
  line L3129 (20.0369, -94.4741) -> (20.012, -94.4275)
  line L3130 (20.012, -94.4275) -> (19.9841, -94.3827)
  line L3131 (19.9841, -94.3827) -> (19.9533, -94.3397)
  line L3132 (19.9533, -94.3397) -> (19.9198, -94.2989)
  line L3133 (19.9198, -94.2989) -> (19.8859, -94.2627)
  line L3134 (19.8859, -94.2627) -> (18.6028, -92.9797)
  arc A198 (18.6028, -92.9797) -> (17.92, -93.2625) centre (18.32, -93.2625) ccw
  line L3135 (17.92, -93.2625) -> (17.92, -95.2997)
  line L3136 (17.92, -95.2997) -> (16.5635, -95.2997)
  line L3137 (16.5635, -95.2997) -> (14.02, -92.7562)
  line L3138 (14.02, -92.7562) -> (14.02, -90.1167)
  line L3139 (14.02, -90.1167) -> (13.903, -89.9997)
  line L3140 (13.903, -89.9997) -> (14.02, -89.8826)
  line L3141 (14.02, -89.8826) -> (14.02, -87.2432)
  line L3142 (14.02, -87.2432) -> (16.5635, -84.6997)
  line L3143 (16.5635, -84.6997) -> (17.92, -84.6997)
  line L3144 (17.92, -84.6997) -> (17.92, -86.7368)
  arc A199 (17.92, -86.7368) -> (18.6028, -87.0197) centre (18.32, -86.7368) ccw
  line L3145 (18.6028, -87.0197) -> (19.8859, -85.7366)
  line L3146 (19.8859, -85.7366) -> (19.9198, -85.7004)
  line L3147 (19.9198, -85.7004) -> (19.9533, -85.6596)
  line L3148 (19.9533, -85.6596) -> (19.9841, -85.6166)
  line L3149 (19.9841, -85.6166) -> (20.012, -85.5718)
  line L3150 (20.012, -85.5718) -> (20.0369, -85.5252)
  line L3151 (20.0369, -85.5252) -> (20.0587, -85.4771)
  line L3152 (20.0587, -85.4771) -> (20.0773, -85.4277)
  line L3153 (20.0773, -85.4277) -> (20.0926, -85.3771)
  line L3154 (20.0926, -85.3771) -> (20.1046, -85.3257)
  line L3155 (20.1046, -85.3257) -> (20.1132, -85.2736)
  line L3156 (20.1132, -85.2736) -> (20.1184, -85.221)
  line L3157 (20.1184, -85.221) -> (20.12, -85.1715)
  line L3158 (20.12, -85.1715) -> (20.12, -81.4997)
  line L3159 (20.12, -81.4997) -> (20.12, -80.4997)
  arc A200 (20.12, -80.4997) -> (19.42, -79.7997) centre (19.42, -80.4997) ccw
  line L3160 (19.42, -79.7997) -> (18.42, -79.7997)
  line L3161 (18.42, -79.7997) -> (14.7482, -79.7997)
  line L3162 (14.7482, -79.7997) -> (14.6987, -79.8013)
  line L3163 (14.6987, -79.8013) -> (14.6461, -79.8065)
  line L3164 (14.6461, -79.8065) -> (14.594, -79.8151)
  line L3165 (14.594, -79.8151) -> (14.5425, -79.8271)
  line L3166 (14.5425, -79.8271) -> (14.492, -79.8424)
  line L3167 (14.492, -79.8424) -> (14.4426, -79.861)
  line L3168 (14.4426, -79.861) -> (14.3945, -79.8828)
  line L3169 (14.3945, -79.8828) -> (14.3479, -79.9077)
  line L3170 (14.3479, -79.9077) -> (14.303, -79.9356)
  line L3171 (14.303, -79.9356) -> (14.2601, -79.9663)
  line L3172 (14.2601, -79.9663) -> (14.2193, -79.9999)
  line L3173 (14.2193, -79.9999) -> (14.1831, -80.0337)
  line L3174 (14.1831, -80.0337) -> (12.9, -81.3168)
  arc A201 (12.9, -81.3168) -> (13.1828, -81.9997) centre (13.1828, -81.5997) ccw
  line L3175 (13.1828, -81.9997) -> (15.22, -81.9997)
  line L3176 (15.22, -81.9997) -> (15.22, -83.3562)
  line L3177 (15.22, -83.3562) -> (12.6765, -85.8997)
  line L3178 (12.6765, -85.8997) -> (10.0441, -85.8997)
  line L3179 (10.0441, -85.8997) -> (9.92, -86.0238)
  line L3180 (16.0765, -97.4997) -> (17.92, -97.4997)
  line L3181 (17.92, -97.4997) -> (17.92, -102.4997)
  line L3182 (17.92, -102.4997) -> (16.0765, -102.4997)
  line L3183 (16.0765, -102.4997) -> (12.6765, -105.8997)
  line L3184 (12.6765, -105.8997) -> (10.0441, -105.8997)
  line L3185 (10.0441, -105.8997) -> (9.92, -106.0238)
  line L3186 (9.92, -106.0238) -> (9.7959, -105.8997)
  line L3187 (9.7959, -105.8997) -> (7.1635, -105.8997)
  line L3188 (7.1635, -105.8997) -> (3.7635, -102.4997)
  line L3189 (3.7635, -102.4997) -> (1.92, -102.4997)
  line L3190 (1.92, -102.4997) -> (1.92, -97.4997)
  line L3191 (1.92, -97.4997) -> (3.7635, -97.4997)
  line L3192 (3.7635, -97.4997) -> (7.1635, -94.0997)
  line L3193 (7.1635, -94.0997) -> (9.7959, -94.0997)
  line L3194 (9.7959, -94.0997) -> (9.92, -93.9755)
  line L3195 (9.92, -93.9755) -> (10.0441, -94.0997)
  line L3196 (10.0441, -94.0997) -> (12.6765, -94.0997)
  line L3197 (12.6765, -94.0997) -> (16.0765, -97.4997)
  line L3198 (9.92, -113.9755) -> (10.0441, -114.0997)
  line L3199 (10.0441, -114.0997) -> (12.6765, -114.0997)
  line L3200 (12.6765, -114.0997) -> (16.0765, -117.4997)
  line L3201 (16.0765, -117.4997) -> (17.92, -117.4997)
  line L3202 (17.92, -117.4997) -> (17.92, -122.4997)
  line L3203 (17.92, -122.4997) -> (16.0765, -122.4997)
  line L3204 (16.0765, -122.4997) -> (12.6765, -125.8997)
  line L3205 (12.6765, -125.8997) -> (10.0441, -125.8997)
  line L3206 (10.0441, -125.8997) -> (9.92, -126.0238)
  line L3207 (9.92, -126.0238) -> (9.7959, -125.8997)
  line L3208 (9.7959, -125.8997) -> (7.1635, -125.8997)
  line L3209 (7.1635, -125.8997) -> (3.7635, -122.4997)
  line L3210 (3.7635, -122.4997) -> (1.92, -122.4997)
  line L3211 (1.92, -122.4997) -> (1.92, -117.4997)
  line L3212 (1.92, -117.4997) -> (3.7635, -117.4997)
  line L3213 (3.7635, -117.4997) -> (7.1635, -114.0997)
  line L3214 (7.1635, -114.0997) -> (9.7959, -114.0997)
  line L3215 (9.7959, -114.0997) -> (9.92, -113.9755)
  line L3216 (-0.2786, -145.2189) -> (-0.2732, -145.2736)
  line L3217 (-0.2732, -145.2736) -> (-0.2646, -145.3257)
  line L3218 (-0.2646, -145.3257) -> (-0.2526, -145.3771)
  line L3219 (-0.2526, -145.3771) -> (-0.2373, -145.4277)
  line L3220 (-0.2373, -145.4277) -> (-0.2187, -145.4771)
  line L3221 (-0.2187, -145.4771) -> (-0.1969, -145.5252)
  line L3222 (-0.1969, -145.5252) -> (-0.172, -145.5718)
  line L3223 (-0.172, -145.5718) -> (-0.1441, -145.6166)
  line L3224 (-0.1441, -145.6166) -> (-0.1133, -145.6596)
  line L3225 (-0.1133, -145.6596) -> (-0.0798, -145.7004)
  line L3226 (-0.0798, -145.7004) -> (-0.0459, -145.7366)
  line L3227 (-0.0459, -145.7366) -> (1.2372, -147.0197)
  arc A202 (1.2372, -147.0197) -> (1.92, -146.7368) centre (1.52, -146.7368) ccw
  line L3228 (1.92, -146.7368) -> (1.92, -144.6997)
  line L3229 (1.92, -144.6997) -> (3.2765, -144.6997)
  line L3230 (3.2765, -144.6997) -> (5.82, -147.2432)
  line L3231 (5.82, -147.2432) -> (5.82, -149.8826)
  line L3232 (5.82, -149.8826) -> (5.937, -149.9997)
  line L3233 (5.937, -149.9997) -> (5.82, -150.1167)
  line L3234 (5.82, -150.1167) -> (5.82, -152.7562)
  line L3235 (5.82, -152.7562) -> (3.2765, -155.2997)
  line L3236 (3.2765, -155.2997) -> (1.92, -155.2997)
  line L3237 (1.92, -155.2997) -> (1.92, -153.2625)
  arc A203 (1.92, -153.2625) -> (1.2372, -152.9797) centre (1.52, -153.2625) ccw
  line L3238 (1.2372, -152.9797) -> (-0.0459, -154.2627)
  line L3239 (-0.0459, -154.2627) -> (-0.0798, -154.2989)
  line L3240 (-0.0798, -154.2989) -> (-0.1133, -154.3397)
  line L3241 (-0.1133, -154.3397) -> (-0.1441, -154.3827)
  line L3242 (-0.1441, -154.3827) -> (-0.172, -154.4275)
  line L3243 (-0.172, -154.4275) -> (-0.1969, -154.4741)
  line L3244 (-0.1969, -154.4741) -> (-0.2187, -154.5222)
  line L3245 (-0.2187, -154.5222) -> (-0.2373, -154.5717)
  line L3246 (-0.2373, -154.5717) -> (-0.2526, -154.6222)
  line L3247 (-0.2526, -154.6222) -> (-0.2646, -154.6736)
  line L3248 (-0.2646, -154.6736) -> (-0.2732, -154.7258)
  line L3249 (-0.2732, -154.7258) -> (-0.2786, -154.7804)
  line L3250 (-0.2786, -154.7804) -> (-0.28, -154.8985)
  line L3251 (-0.28, -154.8985) -> (-0.28, -165.1009)
  line L3252 (-0.28, -165.1009) -> (-0.2786, -165.2189)
  line L3253 (-0.2786, -165.2189) -> (-0.2732, -165.2736)
  line L3254 (-0.2732, -165.2736) -> (-0.2646, -165.3257)
  line L3255 (-0.2646, -165.3257) -> (-0.2526, -165.3771)
  line L3256 (-0.2526, -165.3771) -> (-0.2373, -165.4277)
  line L3257 (-0.2373, -165.4277) -> (-0.2187, -165.4771)
  line L3258 (-0.2187, -165.4771) -> (-0.1969, -165.5252)
  line L3259 (-0.1969, -165.5252) -> (-0.172, -165.5718)
  line L3260 (-0.172, -165.5718) -> (-0.1441, -165.6166)
  line L3261 (-0.1441, -165.6166) -> (-0.1133, -165.6596)
  line L3262 (-0.1133, -165.6596) -> (-0.0798, -165.7004)
  line L3263 (-0.0798, -165.7004) -> (-0.0459, -165.7366)
  line L3264 (-0.0459, -165.7366) -> (1.2372, -167.0197)
  arc A204 (1.2372, -167.0197) -> (1.92, -166.7368) centre (1.52, -166.7368) ccw
  line L3265 (1.92, -166.7368) -> (1.92, -164.6997)
  line L3266 (1.92, -164.6997) -> (3.2765, -164.6997)
  line L3267 (3.2765, -164.6997) -> (5.82, -167.2432)
  line L3268 (5.82, -167.2432) -> (5.82, -169.8826)
  line L3269 (5.82, -169.8826) -> (5.937, -169.9997)
  line L3270 (5.937, -169.9997) -> (5.82, -170.1167)
  line L3271 (5.82, -170.1167) -> (5.82, -172.7562)
  line L3272 (5.82, -172.7562) -> (3.2765, -175.2997)
  line L3273 (3.2765, -175.2997) -> (1.92, -175.2997)
  line L3274 (1.92, -175.2997) -> (1.92, -173.2625)
  arc A205 (1.92, -173.2625) -> (1.2372, -172.9797) centre (1.52, -173.2625) ccw
  line L3275 (1.2372, -172.9797) -> (-0.0459, -174.2627)
  line L3276 (-0.0459, -174.2627) -> (-0.0798, -174.2989)
  line L3277 (-0.0798, -174.2989) -> (-0.1133, -174.3397)
  line L3278 (-0.1133, -174.3397) -> (-0.1441, -174.3827)
  line L3279 (-0.1441, -174.3827) -> (-0.172, -174.4275)
  line L3280 (-0.172, -174.4275) -> (-0.1969, -174.4741)
  line L3281 (-0.1969, -174.4741) -> (-0.2187, -174.5222)
  line L3282 (-0.2187, -174.5222) -> (-0.2373, -174.5717)
  line L3283 (-0.2373, -174.5717) -> (-0.2526, -174.6222)
  line L3284 (-0.2526, -174.6222) -> (-0.2646, -174.6736)
  line L3285 (-0.2646, -174.6736) -> (-0.2732, -174.7258)
  line L3286 (-0.2732, -174.7258) -> (-0.2786, -174.7804)
  line L3287 (-0.2786, -174.7804) -> (-0.28, -174.8985)
  line L3288 (-0.28, -174.8985) -> (-0.28, -185.1009)
  line L3289 (-0.28, -185.1009) -> (-0.2786, -185.2189)
  line L3290 (-0.2786, -185.2189) -> (-0.2732, -185.2736)
  line L3291 (-0.2732, -185.2736) -> (-0.2646, -185.3257)
  line L3292 (-0.2646, -185.3257) -> (-0.2526, -185.3771)
  line L3293 (-0.2526, -185.3771) -> (-0.2373, -185.4277)
  line L3294 (-0.2373, -185.4277) -> (-0.2187, -185.4771)
  line L3295 (-0.2187, -185.4771) -> (-0.1969, -185.5252)
  line L3296 (-0.1969, -185.5252) -> (-0.172, -185.5718)
  line L3297 (-0.172, -185.5718) -> (-0.1441, -185.6166)
  line L3298 (-0.1441, -185.6166) -> (-0.1133, -185.6596)
  line L3299 (-0.1133, -185.6596) -> (-0.0798, -185.7004)
  line L3300 (-0.0798, -185.7004) -> (-0.0459, -185.7366)
  line L3301 (-0.0459, -185.7366) -> (1.2372, -187.0197)
  arc A206 (1.2372, -187.0197) -> (1.92, -186.7368) centre (1.52, -186.7368) ccw
  line L3302 (1.92, -186.7368) -> (1.92, -184.6997)
  line L3303 (1.92, -184.6997) -> (3.2765, -184.6997)
  line L3304 (3.2765, -184.6997) -> (5.82, -187.2432)
  line L3305 (5.82, -187.2432) -> (5.82, -189.8826)
  line L3306 (5.82, -189.8826) -> (5.937, -189.9997)
  line L3307 (5.937, -189.9997) -> (5.82, -190.1167)
  line L3308 (5.82, -190.1167) -> (5.82, -192.7562)
  line L3309 (5.82, -192.7562) -> (3.2765, -195.2997)
  line L3310 (3.2765, -195.2997) -> (1.92, -195.2997)
  line L3311 (1.92, -195.2997) -> (1.92, -193.2625)
  arc A207 (1.92, -193.2625) -> (1.2372, -192.9797) centre (1.52, -193.2625) ccw
  line L3312 (1.2372, -192.9797) -> (-0.0459, -194.2627)
  line L3313 (-0.0459, -194.2627) -> (-0.0798, -194.2989)
  line L3314 (-0.0798, -194.2989) -> (-0.1133, -194.3397)
  line L3315 (-0.1133, -194.3397) -> (-0.1441, -194.3827)
  line L3316 (-0.1441, -194.3827) -> (-0.172, -194.4275)
  line L3317 (-0.172, -194.4275) -> (-0.1969, -194.4741)
  line L3318 (-0.1969, -194.4741) -> (-0.2187, -194.5222)
  line L3319 (-0.2187, -194.5222) -> (-0.2373, -194.5717)
  line L3320 (-0.2373, -194.5717) -> (-0.2526, -194.6222)
  line L3321 (-0.2526, -194.6222) -> (-0.2646, -194.6736)
  line L3322 (-0.2646, -194.6736) -> (-0.2732, -194.7258)
  line L3323 (-0.2732, -194.7258) -> (-0.2786, -194.7804)
  line L3324 (-0.2786, -194.7804) -> (-0.28, -194.8985)
  line L3325 (-0.28, -194.8985) -> (-0.28, -205.1009)
  line L3326 (-0.28, -205.1009) -> (-0.2786, -205.2189)
  line L3327 (-0.2786, -205.2189) -> (-0.2732, -205.2736)
  line L3328 (-0.2732, -205.2736) -> (-0.2646, -205.3257)
  line L3329 (-0.2646, -205.3257) -> (-0.2526, -205.3771)
  line L3330 (-0.2526, -205.3771) -> (-0.2373, -205.4277)
  line L3331 (-0.2373, -205.4277) -> (-0.2187, -205.4771)
  line L3332 (-0.2187, -205.4771) -> (-0.1969, -205.5252)
  line L3333 (-0.1969, -205.5252) -> (-0.172, -205.5718)
  line L3334 (-0.172, -205.5718) -> (-0.1441, -205.6166)
  line L3335 (-0.1441, -205.6166) -> (-0.1133, -205.6596)
  line L3336 (-0.1133, -205.6596) -> (-0.0798, -205.7004)
  line L3337 (-0.0798, -205.7004) -> (-0.0459, -205.7366)
  line L3338 (-0.0459, -205.7366) -> (1.2372, -207.0197)
  arc A208 (1.2372, -207.0197) -> (1.92, -206.7368) centre (1.52, -206.7368) ccw
  line L3339 (1.92, -206.7368) -> (1.92, -204.6997)
  line L3340 (1.92, -204.6997) -> (3.2765, -204.6997)
  line L3341 (3.2765, -204.6997) -> (5.82, -207.2432)
  line L3342 (5.82, -207.2432) -> (5.82, -209.8826)
  line L3343 (5.82, -209.8826) -> (5.937, -209.9997)
  line L3344 (5.937, -209.9997) -> (5.82, -210.1167)
  line L3345 (5.82, -210.1167) -> (5.82, -212.7562)
  line L3346 (5.82, -212.7562) -> (3.2765, -215.2997)
  line L3347 (3.2765, -215.2997) -> (1.92, -215.2997)
  line L3348 (1.92, -215.2997) -> (1.92, -213.2625)
  arc A209 (1.92, -213.2625) -> (1.2372, -212.9797) centre (1.52, -213.2625) ccw
  line L3349 (1.2372, -212.9797) -> (-0.0459, -214.2627)